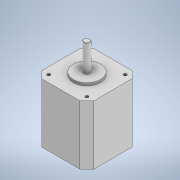
# Autodesk Inventor part: Stepper_NEMA17_48mm
Saved by Autodesk Inventor 2022 (Build 260153000, 153)
## iProperties
Created: 2021-06-15
Part Number: Stepper_NEMA17_48mm
Material: Generic
Document SubType Name: Modeling
Designer: burgessb
Density: 1 g/cm^3
Appearance: Default
Author: burgessb
Autodesk Inventor part; units mm, degrees
ref_plane "YZ Plane" through (0, 0, 0) normal (1, 0, 0) x (0, 1, 0)
ref_plane "XZ Plane" through (0, 0, 0) normal (0, 1, 0) x (-1, 0, 0)
ref_plane "XY Plane" through (0, 0, 0) normal (0, 0, 1) x (1, 0, 0)
sketch "Sketch1" plane through (0, 0, 0) normal (0, 1, 0) x (-1, 0, 0)
  line L0 (-21.15, 21.15) -> (21.15, 21.15)
  line L1 (21.15, 21.15) -> (21.15, -21.15)
  line L2 (21.15, -21.15) -> (-21.15, -21.15)
  line L3 (-21.15, -21.15) -> (-21.15, 21.15)
  line L4 (-21.15, 21.15) -> (21.15, -21.15) construction
  line L5 (21.15, 21.15) -> (-21.15, -21.15) construction
  line L6 (-15.5, 15.5) -> (15.5, 15.5)
  line L7 (15.5, 15.5) -> (15.5, -15.5)
  line L8 (15.5, -15.5) -> (-15.5, -15.5)
  line L9 (-15.5, -15.5) -> (-15.5, 15.5)
  line L10 (-15.5, 15.5) -> (15.5, -15.5) construction
  line L11 (15.5, 15.5) -> (-15.5, -15.5) construction
  line L12 (15.5, -21.15) -> (21.15, -15.5)
  line L13 (-21.15, -15.5) -> (-15.5, -21.15)
  line L14 (-21.15, 15.5) -> (-15.5, 21.15)
  line L15 (15.5, 21.15) -> (21.15, 15.5)
  point P0 (0, 0)
  dimension "d0" = 42.3
  dimension "d1" = 42.3
  dimension "d2" = 31
  dimension "d3" = 31
  dimension "d4" = 31
  dimension "d5" = 31
  dimension "d6" = 31
  dimension "d7" = 31
  dimension "d8" = 45
  constraints: 32 end point, 10 point on line, 4 midpoint, 4 parallel, 3 perpendicular, 2 horizontal
  measures "d0" distance of L1.end L2.end
  measures "d1" distance of L0.end L1.end
  measures "d2" distance of L7.end L8.end
  measures "d3" distance of L6.end L7.end
  measures "d4" distance of L12.end L15.end
  measures "d5" distance of L13.end L12.start
  measures "d6" distance of L14.end L15.start
  measures "d7" distance of L13.start L14.start
  measures "d8" angle of L3 L14
extrude "Extrusion1" add sketch "Sketch1" along normal blind 48 contours L0 L15 L1 L12 L2 L13 L3 L14 | L6 L7 L8 L9
sketch "Sketch2" plane through (0, 48, 0) normal (0, 1, 0) x (1, 0, 0)
  circle A0 centre (0, 0) radius 11
  dimension "d11" = 22
  constraints: 1 centre point, 1 coincident
  measures "d11" diameter of A0
extrude "Extrusion2" add sketch "Sketch2" along normal blind 2
sketch "Sketch3" plane through (0, 50, 0) normal (0, 1, 0) x (1, 0, 0)
  circle A0 centre (0, 0) radius 2.5
  dimension "d14" = 5
  constraints: 1 centre point, 1 coincident
  measures "d14" diameter of A0
extrude "Extrusion3" add sketch "Sketch3" along normal blind 22
sketch "Sketch4" plane through (0, 72, 0) normal (0, 1, 0) x (1, 0, 0)
  circle A0 centre (0, 0) radius 2.5 projected
  line L0 (-1.5, 2) -> (1.5, 2)
  circle A1 centre (0, 0) radius 2.5 projected
  dimension "d21" = 5
  dimension "d20" = 2
  constraints: 2 end point, 1 horizontal, 1 point on circle, 2 other
  measures "d20" distance from line of point (0, 0) L0
extrude "Extrusion4" cut sketch "Sketch4" against normal blind 15 contours L0 A0 picked at (-0.3466, 2.0912)
chamfer "Chamfer2" distance 0.2 angle 45 3 edges at (-1.118, 72, 2.2361) (2.2361, 72, -1.118) (0, 72, -2)
sketch "Sketch5" plane through (0, 48, 0) normal (0, 1, 0) x (1, 0, 0)
  circle A0 centre (0, 0) radius 11 projected
  line L0 (-15.5, -21.15) -> (15.5, -21.15) projected
  line L1 (15.5, -21.15) -> (21.15, -15.5) projected
  line L2 (21.15, -15.5) -> (21.15, 15.5) projected
  line L3 (21.15, 15.5) -> (15.5, 21.15) projected
  line L4 (15.5, 21.15) -> (-15.5, 21.15) projected
  line L5 (-15.5, 21.15) -> (-21.15, 15.5) projected
  line L6 (-21.15, 15.5) -> (-21.15, -15.5) projected
  line L7 (-21.15, -15.5) -> (-15.5, -21.15) projected
  point P0 (-15.5, 15.5)
  point P1 (15.5, 15.5)
  point P2 (-15.5, -15.5)
  point P3 (15.5, -15.5)
  dimension "d29" = 31
  dimension "d32" = 31
  dimension "d35" = 15.5
  dimension "d36" = 15.5
  constraints: 1 horizontal, 1 vertical, 3 other
  measures "d29" distance of point (-15.5, 15.5) point (15.5, 15.5)
  measures "d32" distance of point (-15.5, 15.5) point (-15.5, -15.5)
  measures "d35" horizontal distance of point (0, 0) point (-15.5, 15.5)
  measures "d36" horizontal distance of point (0, 0) point (-15.5, 15.5)
hole "Hole1" at (-15.5, 48, -15.5) at (15.5, 48, -15.5) at (-15.5, 48, 15.5) at (15.5, 48, 15.5) direction (0, -1, 0) diameter 2.459 depth 4.5 tip angle 118 thread size "M3x0.5" class "6H" standard "ANSI Metric M Profile"
sketch "Sketch6" plane through (15.5, 0, -21.15) normal (0, 0, -1) x (-1, 0, 0)
  line L0 (0, 0) -> (31, 0) projected
  line L1 (31, 0) -> (31, 48) projected
  line L2 (0, 48) -> (31, 48) projected
  line L3 (0, 0) -> (0, 48) projected
  line L4 (7.5, 10.5) -> (23.5, 10.5)
  line L5 (23.5, 10.5) -> (23.5, 4.5)
  line L6 (23.5, 4.5) -> (7.5, 4.5)
  line L7 (7.5, 4.5) -> (7.5, 10.5)
  point P0 (15.5, 0)
  dimension "d44" = 16
  dimension "d45" = 6
  dimension "d46" = 10.5
  dimension "d47" = 31
  dimension "d48" = 7.5
  constraints: 8 end point, 2 parallel, 1 horizontal, 1 perpendicular
  measures "d44" distance of L5.end L6.end
  measures "d45" distance of L4.end L5.end
  measures "d46" distance between parallel lines of L0 L4
  measures "d47" distance of L0.start L0.end
  measures "d48" distance between parallel lines of L1 L5
extrude "Extrusion5" add sketch "Sketch6" along normal blind 5 contours L4 L5 L6 L7
equation "\"d35\" = 0.5 * d29"
equation "\"d36\" = 0.5 * d32"
equation "\"d48\" = -0.5 * d44 + 0.5 * d47"
body "Solid1"
